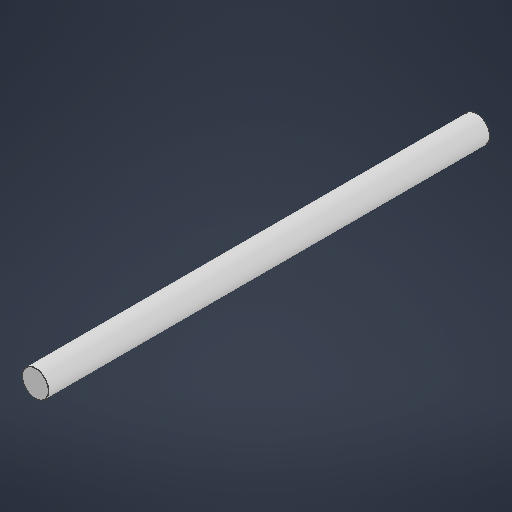
# Autodesk Inventor part: cevirme_kolu
Saved by Autodesk Inventor 2025.4 (Build 294407000, 407)
## iProperties
Created: 2026-06-17
Part Number: cevirme_kolu
Material: Generic
Document SubType Name: Modeling
Designer: yigithan
Density: 1 g/cm^3
Appearance: Default
Author: yigithan
Autodesk Inventor part; units mm, degrees
ref_plane "YZ Plane" through (0, 0, 0) normal (1, 0, 0) x (0, 1, 0)
ref_plane "XZ Plane" through (0, 0, 0) normal (0, 1, 0) x (-1, 0, 0)
ref_plane "XY Plane" through (0, 0, 0) normal (0, 0, 1) x (1, 0, 0)
sketch "Sketch1" plane through (0, 0, 0) normal (0, 0, 1) x (1, 0, 0)
  circle A0 centre (0, 0) radius 3
  dimension "d0" = 6
  constraints: 1 centre point, 1 coincident
  measures "d0" diameter of A0
extrude "Extrusion1" add sketch "Sketch1" along normal blind 100
body "Solid1"
